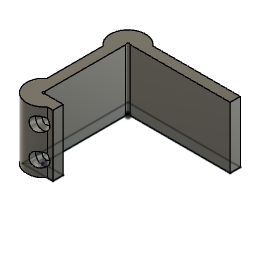
zortrax_fixture_bracket v3 (Autodesk Fusion 360 design; units mm, degrees)
Autodesk Fusion 360 part; units mm, degrees
sketch "Sketch1" plane through (0, 0, 0) normal (0, 1, 0) x (1, 0, 0)
  line L0 (0, 0) -> (0, 53)
  line L1 (0, 0) -> (12.7, 0)
  line L2 (0, 53) -> (63.5, 53)
  line L3 (-6.35, 59.35) -> (63.5, 59.35)
  line L4 (-6.35, -6.35) -> (-6.35, 59.35)
  line L5 (-6.35, -6.35) -> (12.7, -6.35)
  line L6 (12.7, -6.35) -> (12.7, 0)
  line L7 (63.5, 53) -> (63.5, 59.35)
  line L8 (-6.35, -6.35) -> (0.5, 0.5) construction
  line L9 (-6.35, 59.35) -> (0.5, 52.5) construction
  dimension "d1" = 53
  dimension "d2" = 12.7
  dimension "d3" = 63.5
  dimension "d5" = 6.35
  dimension "d6" = 0.5
  dimension "d7" = 0.5
  constraint coincident L0.start L1.start
  constraint vertical L0
  constraint horizontal L1
  constraint perpendicular L0 L2
  constraint perpendicular L1 L6
  constraint coincident L0.start L8
  constraint coincident L0.end L9
  measures "d1" distance of L0.start L0.end
  measures "d2" distance of L0.start L1.end
  measures "d3" distance of L0.end L2.end
  measures "d6" horizontal distance of L0.start L8.end
  measures "d7" horizontal distance of L0.end L9.end
sketch "Sketch2" plane through (0, 0, 0) normal (0, 1, 0) x (1, 0, 0)
  circle A0 centre (0.5, 0.5) radius 1
  circle A1 centre (0.5, 52.5) radius 1
  circle A2 centre (0.5, 52.5) radius 11
  line L0 (-6.35, -6.35) -> (-6.35, 59.35)
  line L1 (-6.35, 59.35) -> (63.5, 59.35)
  line L2 (-6.35, -6.35) -> (12.7, -6.35)
  circle A3 centre (0.5, 0.5) radius 11
  point P0 (0.5, 0.5)
  point P1 (0.5, 52.5)
  dimension "d8" = 2
  dimension "d9" = 22
  constraint coincident P0 A0.centre
  constraint coincident P1 A1.centre
  constraint equal A0 A1
  constraint concentric A0 A3
  constraint equal A2 A3
  measures "d8" diameter of A0
  measures "d9" diameter of A2
ref_plane "WorkPlane1" through (0, 0, 6.35) normal (0, 0, 1) x (1, 0, 0)
sketch "Sketch3" plane through (0, 0, 6.35) normal (0, 0, 1) x (1, 0, 0)
  line L0 (-6.35, 0) -> (12.7, 0)
  line L1 (-6.35, 0) -> (12.7, 0) construction
  line L2 (12.7, 0) -> (12.7, 38.1)
  line L3 (12.7, 38.1) -> (-6.35, 38.1)
  line L4 (-6.35, 38.1) -> (-6.35, 0)
  line L5 (6.35, 0) -> (6.35, 38.1) construction
  line L6 (12.7, 19.05) -> (6.35, 19.05) construction
  circle A0 centre (6.35, 28.575) radius 4.4196
  circle A1 centre (6.35, 9.525) radius 4.4196
  line L7 (0, 0) -> (12.7, 0)
  point P0 (6.35, 9.525)
  point P1 (6.35, 28.575)
  dimension "d11" = 38.1
  dimension "d12" = 19.05
  dimension "d13" = 8.8392
  constraint horizontal L1
  constraint vertical L2
  constraint horizontal L3
  constraint vertical L4
  constraint coincident L0.start L1.start
  constraint coincident L0.end L1.end
  constraint midpoint L2 L6.start
  constraint midpoint L5 L6.end
  constraint coincident L5 P0
  constraint coincident L5 P1
  constraint symmetric L6 P0 P1
  constraint coincident P1 A0.centre
  constraint coincident P0 A1.centre
  constraint equal A0 A1
  constraint vertical L5
  constraint midpoint L5.start L7
  measures "d11" distance of L0.end L2.end
  measures "d12" distance of P0 P1
  measures "d13" diameter of A0
extrude "Extrude1" add sketch "Sketch1" along normal up to surface (38.1 mm away)
extrude "Extrude2" add sketch "Sketch2" along normal up to surface (38.1 mm away) contours A2 L0 L1 | L0 L2 A3 picked at (-6.7442, 49.4093) picked at (-6.7442, 3.5907)
extrude "Extrude3" cut sketch "Sketch3" along normal blind 5 contours A0 | A1
hole "Hole1" at (6.35, 28.575, 6.35) at (6.35, 9.525, 6.35) direction (0, 0, -1) diameter 5.08 depth 25 tip angle 118 countersink diameter 8.8392 countersink angle 82
extrude "Extrude4" cut sketch "Sketch2" along normal up to surface (38.1 mm away) contours A0 | A1
equation "d2 = ( 0.5 * 25.4 ) * 1 mm"
equation "d3 = ( 2.5 * 25.4 ) * 1 mm"
equation "d11 = ( 1.5 * 25.4 ) * 1 mm"
equation "d12 = ( 0.75 * 25.4 ) * 1 mm"
